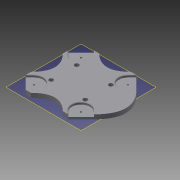
# Autodesk Inventor part: plaque
Saved by Autodesk Inventor 2015 (Build 190159000, 159)
## iProperties
Created: 2015-02-17
Part Number: plaque
Material: Generic
Document SubType Name: Modeling
Designer: Piotr
Density: 1 g/cm^3
Appearance: Default
Mass: 255.612 g
Surface Area: 638.979 cm^2
Volume: 255.612 cm^3
Author: Piotr
Autodesk Inventor part; units mm, degrees
ref_plane "YZ Plane" through (0, 0, 0) normal (1, 0, 0) x (0, 1, 0)
ref_plane "XZ Plane" through (0, 0, 0) normal (0, 1, 0) x (-1, 0, 0)
ref_plane "XY Plane" through (0, 0, 0) normal (0, 0, 1) x (1, 0, 0)
sketch "Sketch2" plane through (0, 0, 0) normal (0, 0, 1) x (1, 0, 0)
  line L0 (-80, 80) -> (80, 80)
  line L1 (80, 80) -> (80, -80)
  line L2 (80, -80) -> (-80, -80)
  line L3 (-80, -80) -> (-80, 80)
  line L4 (157.6027, 0) -> (-257.5856, 0) construction
  line L5 (0, 44.2956) -> (0, -158.1506) construction
  point P0 (0, 0)
  dimension "d0" = 160
  dimension "d1" = 160
  constraints: 12 end point, 2 horizontal, 2 parallel, 2 point on line, 1 perpendicular, 1 vertical, 2 other
  measures "d0" distance of L0.start L0.end
  measures "d1" distance of L0.end L1.end
extrude "Extrusion1" add sketch "Sketch2" along normal blind 10
sketch "Sketch3" plane through (0, 0, 0) normal (0, 0, -1) x (-1, 0, 0)
  line L0 (-80, 50) -> (-50, 80)
  line L1 (-80, 80) -> (80, 80) projected
  line L2 (-80, 80) -> (-80, -80) projected
  line L3 (80, 80) -> (-80, 80) projected
  point P0 (0, 0)
  dimension "d4" = 45
  dimension "d5" = 30
  constraints: 3 point on line, 2 end point
  measures "d4" angle of L1 L0
  measures "d5" horizontal distance of L0.start L0.end
split body "Split1" sketch "Sketch3" result one side removed curves L0 removed pieces at (70, 70, 0.5)
mirror "Mirror1" about plane through (0, 0, 0) normal (0, 1, 0) of "Split1"
mirror "Mirror2" about plane through (0, 0, 0) normal (1, 0, 0) of "Split1", "Mirror1"
sketch "Sketch4" plane through (0, 0, 10) normal (0, 0, 1) x (1, 0, 0)
  line L0 (80, 50) -> (70, 40)
  line L1 (80, 50) -> (50, 80) projected
  line L2 (70, 40) -> (5.0224, 104.9776) construction
  arc A0 (40, 70) -> (70, 40) centre (55, 55) ccw
  line L3 (50, 80) -> (40, 70)
  line L4 (50, 80) -> (80, 50)
  point P0 (0, 0)
  dimension "d17" = 10
  constraints: 8 end point, 2 parallel, 2 perpendicular, 2 point on circle, 2 point on line, 1 centre point
  measures "d17" horizontal distance of L0.start L0.end
extrude "Extrusion2" cut sketch "Sketch4" against normal blind 5
sketch "Sketch5" plane through (0, 0, 5) normal (0, 0, 1) x (1, 0, 0)
  circle A0 centre (55, 55) radius 2
  arc A1 (40, 70) -> (70, 40) centre (55, 55) ccw projected
  point P0 (0, 0)
  dimension "d9" = 4
  constraints: 1 centre point, 1 concentric
  measures "d9" diameter of A0
hole "Hole1" at (55, 55, 5) direction (0, 0, -1) diameter 4 end through all
mirror "Mirror3" about plane through (0, 0, 0) normal (0, 1, 0) of "Extrusion2", "Hole1"
mirror "Mirror4" about plane through (0, 0, 0) normal (1, 0, 0) of "Extrusion2", "Hole1", "Mirror3"
sketch "Sketch6" plane through (0, 0, 10) normal (0, 0, 1) x (1, 0, 0)
  circle A0 centre (40, 30) radius 5
  point P0 (0, 0)
  dimension "d18" = 30
  dimension "d19" = 40
  dimension "d20" = 10
  constraints: 1 centre point
  measures "d18" vertical distance of point (0, 0) A0.centre
  measures "d19" horizontal distance of point (0, 0) A0.centre
  measures "d20" diameter of A0
extrude "Extrusion3" cut sketch "Sketch6" against normal blind 8.5
hole "Hole2" at (40, 30, 1.5) direction (0, 0, -1) diameter 7 end through all
mirror "Mirror5" about plane through (0, 0, 0) normal (0, 1, 0) of "Hole2", "Extrusion3"
mirror "Mirror6" about plane through (0, 0, 0) normal (1, 0, 0) of "Hole2", "Extrusion3", "Mirror5"
sketch "Sketch7" plane through (0, 0, 10) normal (0, 0, 1) x (1, 0, 0)
  line L0 (-80, 50) -> (-80, -50) projected
  line L1 (-80, 37.2721) -> (-42.7279, 0) construction
  line L2 (-42.7279, 0) -> (-80, -37.2721) construction
  spline S0 degree 2 poles (-80, 37.2721) (-42.7279, 0) (-80, -37.2721) knots 1 1 1 2 2 2
  line L3 (-58.7752, 0) -> (-112.5381, 0) construction
  line L4 (-70, 40) -> (-80, 50) projected
  point P0 (0, 0)
  dimension "d50" = 9
  constraints: 4 point on line, 2 end point, 1 horizontal, 1 symmetric about line, 3 other
  measures "d50" distance between parallel lines of L1 L4
extrude "Extrusion4" cut sketch "Sketch7" against normal blind 10
sketch "Sketch9" plane through (0, 0, 10) normal (0, 0, 1) x (1, 0, 0)
  line L0 (-50, -80) -> (50, -80) construction
  line L1 (-37.2721, -80) -> (0, -42.7279) construction
  line L2 (0, -42.7279) -> (37.2721, -80) construction
  spline S0 degree 2 poles (-37.2721, -80) (0, -42.7279) (37.2721, -80) knots 1 1 1 2 2 2
  line L3 (-37.2721, -80) -> (37.2721, -80)
  line L4 (50, -80) -> (-50, -80) projected
  line L5 (-40, -70) -> (-50, -80) projected
  line L6 (50, -80) -> (40, -70) projected
  point P0 (0, 0)
  dimension "d51" = 9
  dimension "d52" = 9
  constraints: 2 end point, 2 point on line, 1 collinear, 3 other
  measures "d51" distance between parallel lines of L1 L5
  measures "d52" distance between parallel lines of L2 L6
extrude "Extrusion5" cut sketch "Sketch9" against normal blind 10
mirror "Mirror8" about plane through (0, 0, 0) normal (0, 1, 0) of "Extrusion5"
ref_plane "Work Plane1" through (80, -50, 0) normal (0, 0, -1) x (-1, 0, 0)
sketch "Sketch10" plane through (80, -50, 0) normal (0, 0, -1) x (-1, 0, 0)
  line L0 (0, 100) -> (-50, 50) construction
  line L1 (-50, 50) -> (0, 0) construction
  spline S0 degree 2 poles (0, 100) (-50, 50) (0, 0) knots 1 1 1 2 2 2
  line L2 (30, 130) -> (0, 100) construction
  line L3 (0, 0) -> (30, -30) construction
  line L4 (0, 100) -> (0, 0)
  line L5 (0, 100) -> (0, 0) projected
  point P0 (80, 50)
  constraints: 3 collinear, 2 end point, 3 other
extrude "Extrusion6" add sketch "Sketch10" against normal up to surface (10 mm away)
chamfer "Chamfer4" distance 1 angle 45 12 edges at (40, 40, 10) (45, 75, 10) (75, 45, 10) (-40, 40, 10) (-75, 45, 10) (-45, 75, 10) (-40, -40, 10) (-45, -75, 10) (-75, -45, 10) (40, -40, 10) (75, -45, 10) (45, -75, 10)
body "Solid1"
